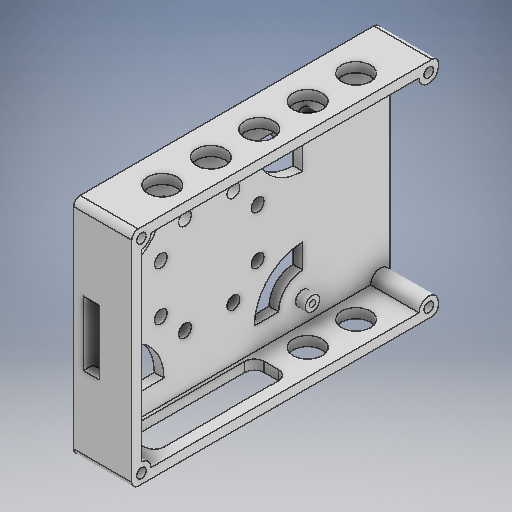
# Autodesk Inventor part: RP5_case
Saved by Autodesk Inventor 2026.1 (Build 301233000, 233)
## iProperties
Created: 2025-12-08
Part Number: RP5_case
Material: Generic
Document SubType Name: Modeling
Designer: emanuel
Density: 1 g/cm^3
Appearance: Default
Author: emanuel
Autodesk Inventor part; units mm, degrees
ref_plane "YZ Plane" through (0, 0, 0) normal (1, 0, 0) x (0, 1, 0)
ref_plane "XZ Plane" through (0, 0, 0) normal (0, 1, 0) x (-1, 0, 0)
ref_plane "XY Plane" through (0, 0, 0) normal (0, 0, 1) x (1, 0, 0)
sketch "Sketch1" plane through (0, 0, 0) normal (1, 0, 0) x (0, 1, 0)
  line L0 (0, 0) -> (49, 0)
  line L1 (49, 0) -> (49, -58)
  line L2 (49, -58) -> (0, -58)
  line L3 (0, -58) -> (0, 0)
  circle A0 centre (49, 0) radius 1
  circle A1 centre (49, -58) radius 1
  circle A2 centre (0, -58) radius 1
  circle A3 centre (0, 0) radius 1
  line L4 (49, 0) -> (49, 7)
  line L5 (49, 7) -> (56, 7)
  line L6 (0, 0) -> (-7, 0)
  line L7 (56, 7) -> (56, -85)
  line L8 (56, 7) -> (-7, 7)
  line L9 (-7, 7) -> (-7, -85)
  line L10 (-7, -85) -> (56, -85)
  line L11 (56, -85) -> (56, 7)
  line L12 (49, 0) -> (52.5, 0)
  line L13 (52.5, 0) -> (52.5, 3.5)
  line L14 (52.5, 3.5) -> (49, 3.5)
  line L15 (49, 3.5) -> (49, 0)
  line L16 (52.5, 3.5) -> (-3.5, 3.5)
  line L17 (-3.5, 3.5) -> (-3.5, -81.5)
  line L18 (-3.5, -81.5) -> (52.5, -81.5)
  line L19 (52.5, -81.5) -> (52.5, 3.5)
  line L20 (56, 7) -> (59, 7)
  line L21 (59, 7) -> (59, 10)
  line L22 (59, 10) -> (56, 10)
  line L23 (56, 10) -> (56, 7)
  line L24 (-7, -85) -> (-10, -85)
  line L25 (-10, -85) -> (-10, -82)
  line L26 (-10, -82) -> (-7, -82)
  line L27 (-7, -82) -> (-7, -85)
  line L28 (59, 10) -> (-10, 10)
  line L29 (-10, 10) -> (-10, -85)
  line L30 (-10, -85) -> (59, -85)
  line L31 (59, -85) -> (59, 10)
  dimension "d0" = 49
  dimension "d1" = 58
  dimension "d2" = 2
  dimension "d3" = 2
  dimension "d4" = 2
  dimension "d5" = 2
  dimension "d6" = 7
  dimension "d7" = 7
  dimension "d8" = 7
  dimension "d9" = 92
  dimension "d10" = 3.5
  dimension "d11" = 3.5
  dimension "d12" = 56
  dimension "d13" = 85
  dimension "d14" = 3
  dimension "d15" = 3
  dimension "d16" = 3
  dimension "d17" = 3
  constraints: 64 end point, 14 parallel, 8 horizontal, 7 perpendicular, 4 centre point, 4 coincident, 2 vertical, 1 point on line
  measures "d0" distance of L1.end L2.end
  measures "d1" distance of L0.end L1.end
  measures "d2" diameter of A0
  measures "d3" diameter of A1
  measures "d4" diameter of A2
  measures "d5" diameter of A3
  measures "d6" distance of L4.start L4.end
  measures "d7" distance of L4.end L5.end
  measures "d8" distance of L6.start L6.end
  measures "d9" distance of L5.end L7.end
  measures "d10" distance of L14.end L13.end
  measures "d11" distance of L13.end L12.end
  measures "d12" distance of L18.end L17.end
  measures "d13" distance of L17.end L16.end
  measures "d14" distance of L22.end L21.end
  measures "d15" distance of L21.end L20.end
  measures "d16" distance of L25.end L26.end
  measures "d17" distance of L24.end L25.end
extrude "Extrusion1" add sketch "Sketch1" along normal blind 3 contours A3 L6 L17 L16 L4 A0 L0 | L0 A0 L1 A1 L2 A2 L3 A3 | L3 A2 L2 A1 L1 A0 L12 L19 L18 L17 L6 A3 | L17 L18 L19 L13 L14 L4 L5 L7 L10 L9 L6 | L6 L9 L8 L4 L16 L17 | L4 L14 L13 L12 A0 | L9 L26 L29 L28 L23 L5 L8 | L9 L24 L25 L26 | L20 L31 L30 L7 | L23 L22 L21 L20
sketch "Sketch2" plane through (3, 0, 0) normal (1, 0, 0) x (0, 0, -1)
  circle A0 centre (0, 49) radius 1 projected
  circle A1 centre (0, 49) radius 2.25
  circle A2 centre (58, 49) radius 1 projected
  circle A3 centre (58, 49) radius 2.25
  circle A4 centre (0, 0) radius 1 projected
  circle A5 centre (0, 0) radius 2.25
  circle A6 centre (58, 0) radius 1 projected
  circle A7 centre (58, 0) radius 2.25
  circle A8 centre (0, 49) radius 1
  circle A9 centre (58, 49) radius 1
  circle A10 centre (0, 0) radius 1
  circle A11 centre (58, 0) radius 1
  line L0 (85, 59) -> (-10, 59) projected
  line L1 (-10, 59) -> (-7, 59)
  line L2 (-7, 59) -> (-7, 56)
  line L3 (-7, 56) -> (-10, 56)
  line L4 (-10, 56) -> (-10, 59)
  line L5 (-10, -10) -> (85, -10) projected
  line L6 (85, -10) -> (82, -10)
  line L7 (82, -10) -> (82, -7)
  line L8 (82, -7) -> (85, -7)
  line L9 (85, -7) -> (85, -10)
  line L10 (-7, 56) -> (82, 56)
  line L11 (82, 56) -> (82, -7)
  line L12 (82, -7) -> (-7, -7)
  line L13 (-7, -7) -> (-7, 56)
  line L14 (-10, 59) -> (-10, -10)
  line L15 (-10, 59) -> (-10, -10) projected
  line L16 (-10, 24.5) -> (-7, 24.5)
  line L17 (-18.5, 34.5) -> (1.5, 34.5)
  line L18 (1.5, 34.5) -> (1.5, 14.5)
  line L19 (1.5, 14.5) -> (-18.5, 14.5)
  line L20 (-18.5, 14.5) -> (-18.5, 34.5)
  line L21 (-18.5, 34.5) -> (1.5, 14.5) construction
  line L22 (1.5, 34.5) -> (-18.5, 14.5) construction
  line L23 (-10, 59) -> (85, 59)
  line L24 (85, 59) -> (85, -10)
  line L25 (85, -10) -> (-10, -10)
  line L26 (-10, -10) -> (-10, 59)
  line L27 (82, 56) -> (85, 56)
  point P0 (-8.5, 24.5)
  point P1 (-7, 14.5)
  point P2 (-10, 14.5)
  point P3 (-10, 34.5)
  point P4 (-7, 34.5)
  dimension "d20" = 4.5
  dimension "d21" = 4.5
  dimension "d22" = 4.5
  dimension "d23" = 4.5
  dimension "d24" = 3
  dimension "d25" = 3
  dimension "d26" = 3
  dimension "d27" = 3
  dimension "d28" = 20
  dimension "d29" = 20
  constraints: 50 end point, 10 parallel, 8 centre point, 8 coincident, 6 perpendicular, 5 horizontal, 5 midpoint, 1 concentric, 1 point on line, 1 vertical
  measures "d20" diameter of A1
  measures "d21" diameter of A3
  measures "d22" diameter of A5
  measures "d23" diameter of A7
  measures "d24" distance of L2.end L3.end
  measures "d25" distance of L1.end L2.end
  measures "d26" distance of L7.end L8.end
  measures "d27" distance of L6.end L7.end
  measures "d28" distance of L18.end L19.end
  measures "d29" distance of L17.end L18.end
extrude "Extrusion2" add sketch "Sketch2" along normal blind 5 contours L24 L27 L10 L2 L0 | L2 L3 L4 L0 | L13 L17 L14 L3 | L9 L5 L7 L8 | L7 L5 L14 L19 L13 L12
extrude "Extrusion3" add sketch "Sketch2" along normal blind 3 contours A1 | A3 | A5 | A7
sketch "Sketch3" plane through (8, 0, 0) normal (1, 0, 0) x (0, 0, -1)
  line L0 (85, 59) -> (-10, 59) projected
  line L1 (85, -10) -> (85, 59) projected
  line L2 (-10, 59) -> (85, 59)
  line L3 (85, 59) -> (85, -10)
  line L4 (85, -10) -> (-10, -10)
  line L5 (-10, -10) -> (-10, 59)
  line L6 (85, 56) -> (-7, 56) projected
  line L7 (-7, -7) -> (85, -7) projected
  line L8 (-7, 56) -> (85, 56)
  line L9 (85, 56) -> (85, -7)
  line L10 (85, -7) -> (-7, -7)
  line L11 (-7, -7) -> (-7, 56)
  point P0 (0, 0)
  constraints: 16 end point, 4 parallel, 2 horizontal, 2 perpendicular
extrude "Extrusion4" add sketch "Sketch3" along normal blind 10 contours L1 L6 L11 L7 L4 L5 L0
fillet "Fillet1" radius 2 4 edges at (9, 59, 10) (9, -10, 10) (9, -10, -85) (9, 59, -85)
fillet "Fillet2" radius 3 2 edges at (10.5, 56, 7) (10.5, -7, 7) inverted yes
sketch "Sketch5" plane through (3, 0, 0) normal (1, 0, 0) x (0, 0, -1)
  line L0 (85, -7) -> (-4, -7) projected
  line L1 (85, -10) -> (82, -10)
  line L2 (82, -10) -> (82, -7)
  line L3 (82, -7) -> (85, -7)
  line L4 (85, -7) -> (85, -10)
  line L5 (85, 59) -> (82, 59)
  line L6 (82, 59) -> (82, 56)
  line L7 (82, 56) -> (85, 56)
  line L8 (85, 56) -> (85, 59)
  circle A0 centre (82, 56) radius 3
  circle A1 centre (82, -7) radius 3
  point P0 (0, 0)
  point P1 (79, -7)
  dimension "d42" = 3
  dimension "d43" = 3
  dimension "d44" = 3
  constraints: 16 end point, 4 parallel, 2 coincident, 2 horizontal, 2 perpendicular, 2 point on line, 6 other
  measures "d42" distance of L2.end L3.end
  measures "d43" distance of L7.end L6.end
  measures "d44" distance of L6.end L5.end
extrude "Extrusion6" add sketch "Sketch5" along normal up to surface (15 mm away) contours L0 A1 | L6 L7 A0 picked at (83.9694, 55.7545)
sketch "Sketch4" plane through (18, 0, 0) normal (1, 0, 0) x (0, 0, -1)
  arc A0 (-7, 53) -> (-4, 56) centre (-7, 56) ccw projected
  circle A1 centre (-7, 56) radius 1.5
  arc A2 (-4, -7) -> (-7, -4) centre (-7, -7) ccw projected
  circle A3 centre (-7, -7) radius 1.5
  arc A4 (79, 56) -> (85, 56) centre (82, 56) ccw projected
  circle A5 centre (82, 56) radius 1.5
  arc A6 (85, -7) -> (79, -7) centre (82, -7) ccw projected
  circle A7 centre (82, -7) radius 1.5
  point P0 (0, 0)
  dimension "d38" = 3
  dimension "d39" = 3
  dimension "d47" = 3
  dimension "d48" = 3
  constraints: 4 centre point, 4 coincident
  measures "d38" diameter of A1
  measures "d39" diameter of A3
  measures "d47" diameter of A5
  measures "d48" diameter of A7
extrude "Extrusion5" cut sketch "Sketch4" against normal blind 5
sketch "Sketch6" plane through (3, 0, 0) normal (1, 0, 0) x (0, 0, -1)
  circle A0 centre (0, 49) radius 1 projected
  circle A1 centre (58, 0) radius 1 projected
  line L0 (0, 49) -> (58, 49)
  line L1 (58, 49) -> (58, 0)
  line L2 (58, 0) -> (0, 0)
  line L3 (0, 0) -> (0, 49)
  line L4 (29, 49) -> (29, 0)
  line L5 (0, 24.5) -> (58, 24.5)
  line L6 (21.5, 29.5) -> (36.5, 29.5)
  line L7 (36.5, 29.5) -> (36.5, 19.5)
  line L8 (36.5, 19.5) -> (21.5, 19.5)
  line L9 (21.5, 19.5) -> (21.5, 29.5)
  line L10 (21.5, 29.5) -> (36.5, 19.5) construction
  line L11 (36.5, 29.5) -> (21.5, 19.5) construction
  line L12 (14, 32) -> (44, 32)
  line L13 (44, 32) -> (44, 17)
  line L14 (44, 17) -> (14, 17)
  line L15 (14, 17) -> (14, 32)
  line L16 (14, 32) -> (44, 17) construction
  line L17 (44, 32) -> (14, 17) construction
  line L18 (21.5, 9.5) -> (36.5, 9.5)
  line L19 (36.5, 9.5) -> (36.5, 39.5)
  line L20 (36.5, 39.5) -> (21.5, 39.5)
  line L21 (21.5, 39.5) -> (21.5, 9.5)
  line L22 (21.5, 9.5) -> (36.5, 39.5) construction
  line L23 (36.5, 9.5) -> (21.5, 39.5) construction
  circle A2 centre (21.5, 39.5) radius 2
  circle A3 centre (36.5, 39.5) radius 2
  circle A4 centre (44, 32) radius 2
  circle A5 centre (44, 17) radius 2
  circle A6 centre (36.5, 9.5) radius 2
  circle A7 centre (21.5, 9.5) radius 2
  circle A8 centre (14, 17) radius 2
  circle A9 centre (14, 32) radius 2
  circle A10 centre (58, 49) radius 15
  circle A11 centre (0, 49) radius 15
  circle A12 centre (0, 0) radius 1 projected
  circle A13 centre (0, 0) radius 15
  circle A14 centre (58, 0) radius 15
  circle A15 centre (58, 49) radius 1 projected
  circle A16 centre (58, 49) radius 7.5
  circle A17 centre (0, 49) radius 7.5
  circle A18 centre (0, 0) radius 7.5
  circle A19 centre (58, 0) radius 7.5
  circle A20 centre (58, 24.5) radius 15
  circle A21 centre (58, 24.5) radius 7.5
  line L24 (58, 24.5) -> (76.2902, 24.5)
  line L25 (76.2902, 24.5) -> (76.2902, 17)
  line L26 (76.2902, 17) -> (58, 17)
  line L27 (58, 17) -> (58, 24.5)
  line L28 (58, 24.5) -> (76.2902, 24.5)
  line L29 (76.2902, 24.5) -> (76.2902, 32)
  line L30 (76.2902, 32) -> (58, 32)
  line L31 (58, 32) -> (58, 24.5)
  point P0 (29, 24.5)
  point P1 (29, 24.5)
  point P2 (0, 7.5)
  point P3 (7.5, 0)
  point P4 (15, 0)
  point P5 (0, 15)
  point P6 (43, 0)
  point P7 (50.5, 0)
  point P8 (58, 7.5)
  point P9 (58, 15)
  point P10 (70.9904, 32)
  point P11 (70.9904, 17)
  point P12 (58, 41.5)
  point P13 (50.5, 49)
  point P14 (43, 49)
  point P15 (58, 34)
  point P16 (7.5, 49)
  point P17 (0, 41.5)
  point P18 (0, 34)
  point P19 (15, 49)
  dimension "d49" = 15
  dimension "d50" = 10
  dimension "d51" = 30
  dimension "d52" = 15
  dimension "d53" = 15
  dimension "d54" = 30
  dimension "d55" = 4
  dimension "d57" = 4
  dimension "d58" = 4
  dimension "d59" = 4
  dimension "d60" = 4
  dimension "d61" = 4
  dimension "d62" = 4
  dimension "d63" = 4
  dimension "d64" = 30
  dimension "d65" = 30
  dimension "d66" = 30
  dimension "d67" = 30
  dimension "d68" = 15
  dimension "d69" = 15
  dimension "d70" = 15
  dimension "d71" = 15
  dimension "d72" = 30
  dimension "d73" = 15
  dimension "d74" = 7.5
  dimension "d75" = 7.5
  constraints: 64 end point, 18 centre point, 18 coincident, 12 midpoint, 12 parallel, 6 horizontal, 6 perpendicular, 1 point on line
  measures "d49" distance of L7.end L8.end
  measures "d50" distance of L6.end L7.end
  measures "d51" distance of L13.end L14.end
  measures "d52" distance of L12.end L13.end
  measures "d53" distance of L20.end L19.end
  measures "d54" distance of L19.end L18.end
  measures "d55" diameter of A2
  measures "d57" diameter of A3
  measures "d58" diameter of A4
  measures "d59" diameter of A5
  measures "d60" diameter of A6
  measures "d61" diameter of A7
  measures "d62" diameter of A8
  measures "d63" diameter of A9
  measures "d64" diameter of A11
  measures "d65" diameter of A10
  measures "d66" diameter of A13
  measures "d67" diameter of A14
  measures "d68" diameter of A16
  measures "d69" diameter of A17
  measures "d70" diameter of A18
  measures "d71" diameter of A19
  measures "d72" diameter of A20
  measures "d73" diameter of A21
  measures "d74" distance of L24.end L25.end
  measures "d75" distance of L29.end L28.end
extrude "Extrusion7" cut sketch "Sketch6" against normal blind 10 contours L0 A11 L3 A17 | L0 A16 L1 A20 A10 | A13 L2 A18 L3 | A20 L1 A10 | A3 L19 L20 | L20 L19 A3 | A2 L21 L20 | L20 L21 A2 | A8 L14 L15 | L15 L14 A8 | A9 L12 L15 | L15 L12 A9 | A20 A4 L13 L12 | A4 A20 | L12 L13 A4 | A14 A20 L1 A19 L2 | A14 L1 A20 | A7 L21 L18 | L18 L21 A7 | A6 L19 L18 | L18 L19 A6 | A20 A5 | A5 L14 L13 A20 | A5 L13 L14 picked at (12.312, 47.3311) picked at (50.2819, 40.5754) picked at (11.6319, 4.3667) picked at (56.9819, 37.5619) picked at (50.2819, 8.4246) picked at (56.9819, 11.4381)
sketch "Sketch7" plane through (0, -10, -83) normal (0, -1, 0) x (1, 0, 0)
  line L0 (0, 91) -> (0, 93) projected
  line L1 (0, 93) -> (10, 93)
  line L2 (10, 93) -> (10, 75.5)
  line L3 (10, 75.5) -> (10, 60.5)
  line L4 (10, 60.5) -> (10, 45.5)
  line L5 (10, 45.5) -> (10, 30.5)
  line L6 (10, 30.5) -> (10, 15.5)
  line L7 (10, 15.5) -> (10, 0.5)
  circle A0 centre (10, 75.5) radius 4.5
  circle A1 centre (10, 60.5) radius 4.5
  circle A2 centre (10, 45.5) radius 4.5
  circle A3 centre (10, 30.5) radius 4.5
  circle A4 centre (10, 15.5) radius 4.5
  point P0 (0, 83)
  dimension "d78" = 10
  dimension "d79" = 17.5
  dimension "d80" = 15
  dimension "d81" = 15
  dimension "d82" = 15
  dimension "d83" = 15
  dimension "d84" = 15
  dimension "d85" = 9
  dimension "d86" = 9
  dimension "d87" = 9
  dimension "d88" = 9
  dimension "d89" = 9
  constraints: 14 end point, 5 centre point, 5 coincident, 5 point on line, 1 horizontal, 1 perpendicular
  measures "d78" distance of L0.end L1.end
  measures "d79" distance of L1.end L2.end
  measures "d80" distance of L2.end L3.end
  measures "d81" distance of L3.end L4.end
  measures "d82" distance of L4.end L5.end
  measures "d83" distance of L5.end L6.end
  measures "d84" distance of L6.end L7.end
  measures "d85" diameter of A0
  measures "d86" diameter of A1
  measures "d87" diameter of A2
  measures "d88" diameter of A3
  measures "d89" diameter of A4
extrude "Extrusion8" cut sketch "Sketch7" against normal up to surface (69 mm away)
sketch "Sketch8" plane through (0, -10, -83) normal (0, -1, 0) x (1, 0, 0)
  circle A0 centre (10, 75.5) radius 4.5 projected
  line L0 (10, 75.5) -> (14.5, 75.5)
  line L1 (14.5, 75.5) -> (14.5, 82.5)
  line L2 (14.5, 82.5) -> (10, 82.5)
  line L3 (10, 82.5) -> (10, 75.5)
  line L4 (10, 75.5) -> (4, 75.5)
  line L5 (4, 75.5) -> (4, 69.5)
  line L6 (4, 69.5) -> (10, 69.5)
  line L7 (10, 69.5) -> (10, 75.5)
  circle A1 centre (10, 60.5) radius 4.5 projected
  circle A2 centre (10, 45.5) radius 4.5 projected
  line L8 (10, 60.5) -> (14.3875, 60.5)
  line L9 (14.3875, 60.5) -> (14.3875, 46.5)
  line L10 (14.3875, 46.5) -> (10, 46.5)
  line L11 (10, 46.5) -> (10, 60.5)
  line L12 (10, 46.5) -> (4, 46.5)
  line L13 (4, 46.5) -> (4, 41)
  line L14 (4, 41) -> (10, 41)
  line L15 (10, 41) -> (10, 46.5)
  line L16 (4, 41) -> (14.5, 41)
  line L17 (14.5, 41) -> (14.5, 82.5)
  line L18 (14.5, 82.5) -> (4, 82.5)
  line L19 (4, 82.5) -> (4, 41)
  point P0 (0, 83)
  point P1 (10, 41)
  point P2 (10, 41)
  point P3 (14.5, 45.5)
  point P4 (14.5, 45.5)
  point P5 (14.3875, 59.5)
  point P6 (14.5, 60.5)
  point P7 (14.5, 60.5)
  dimension "d92" = 7
  dimension "d93" = 6
  dimension "d94" = 6
  dimension "d98" = 41.5
  constraints: 40 end point, 10 parallel, 5 horizontal, 5 perpendicular, 2 other
  measures "d92" distance of L1.end L0.end
  measures "d93" distance of L6.end L5.end
  measures "d94" distance of L5.end L4.end
  measures "d98" distance of L16.end L1.end
extrude "Extrusion9" cut sketch "Sketch8" against normal blind 5 contours L17 A1 L11 A2 L12 L19 L6 L7 A0 | A0 L3 L2 L1 | A0 L4 L19 L18 L3 | L7 L6 L5 L4 A0 | A1 L9 A2 L11 | L17 L16 A2 | L14 L13 L12 A2
fillet "Fillet3" radius 3 4 edges at (14.5, -8.5, -0.5) (4, -8.5, -0.5) (4, -8.5, -42) (14.5, -8.5, -42)
body "Solid1"
